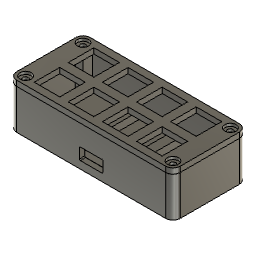
macropad v4 (Autodesk Fusion 360 design; units mm, degrees)
Autodesk Fusion 360 part; units mm, degrees
sketch "Sketch1" plane through (0, 0, 0) normal (0, 0, 1) x (1, 0, 0)
  line L0 (0, 1.7577) -> (18, 1.7577)
  line L1 (18, 1.7577) -> (18, -32.1423)
  line L2 (18, -32.1423) -> (0, -32.1423)
  line L3 (0, -32.1423) -> (0, 1.7577)
  line L4 (4.4, 2.6577) -> (13.6, 2.6577)
  line L5 (13.6, 2.6577) -> (13.6, -4.8423)
  line L6 (13.6, -4.8423) -> (4.4, -4.8423)
  line L7 (4.4, -4.8423) -> (4.4, 2.6577)
  dimension "d1" = 18
  dimension "d2" = 33.9
  dimension "d3" = 9.2
  dimension "d4" = 7.5
  dimension "d5" = 0.9
  dimension "d6" = 4.4
  dimension "d7" = 4.4
  constraint horizontal L0
  constraint vertical L1
  constraint horizontal L2
  constraint vertical L3
  constraint horizontal L4
  constraint vertical L5
  constraint horizontal L6
  constraint vertical L7
  measures "d1" distance of L0.start L0.end
  measures "d2" distance of L0.start L2.end
  measures "d3" distance of L4.start L4.end
  measures "d4" distance of L4.start L6.end
  measures "d5" distance of L0 L4
  measures "d6" distance of L1 L5
  measures "d7" distance of L3 L7
extrude "Extrude1" add sketch "Sketch1" against normal blind 1.75 contours L0 L1 L2 L3 L5 L6 L7 | L0 L5 L6 L7 makes body 1
extrude "Extrude2" add sketch "Sketch1" along normal blind 3.2 contours L0 L4 L5 L7 | L0 L5 L6 L7 bodies 1
fillet "Fillet1" radius 1 2 edges at (13.6, -1.0923, 3.2) (4.4, -1.0923, 3.2) on bodies 1
fillet "Fillet2" radius 1 2 edges at (13.6, 2.2077, 0) (4.4, 2.2077, 0) on bodies 1
sketch "Sketch2" plane through (0, 0, 0) normal (0, 0, 1) x (1, 0, 0)
  line L0 (0, 0) -> (-15.86, 0)
  line L1 (-15.86, 0) -> (-15.86, 15.86)
  line L2 (-15.86, 15.86) -> (0, 15.86)
  line L3 (0, 15.86) -> (0, 0)
  line L4 (-0.88, 14.98) -> (-14.98, 14.98)
  line L5 (-14.98, 14.98) -> (-14.98, 0.88)
  line L6 (-14.98, 0.88) -> (-0.88, 0.88)
  line L7 (-0.88, 0.88) -> (-0.88, 14.98)
  line L8 (-0.88, 14.98) -> (-14.98, 0.88) construction
  line L9 (-14.98, 14.98) -> (-0.88, 0.88) construction
  point P0 (-7.93, 7.93)
  dimension "d16" = 15.86
  dimension "d17" = 15.86
  dimension "d18" = 14.1
  dimension "d19" = 14.1
  dimension "d26" = 0.88
  dimension "d27" = 0.88
  dimension "d28" = 0.88
  dimension "d29" = 0.88
  constraint horizontal L0
  constraint vertical L1
  constraint horizontal L2
  constraint vertical L3
  constraint coincident L0.start L3.end
  constraint horizontal L4
  constraint perpendicular L4 L5
  constraint parallel L4 L6
  constraint parallel L5 L7
  constraint coincident L8 P0
  constraint coincident L9 P0
  measures "d16" distance of L0.start L0.end
  measures "d17" distance of L0.start L2.end
  measures "d18" distance of L5.end L6.end
  measures "d19" distance of L4.end L5.end
  measures "d26" distance of L1 L5
  measures "d27" distance of L3 L7
  measures "d28" distance of L0 L6
  measures "d29" distance of L2 L4
extrude "Extrude3" add sketch "Sketch2" along normal blind 1 separate body contours L0 L1 L2 L3 | L4 L5 L6 L7 makes body 2
extrude "Extrude4" add sketch "Sketch2" against normal blind 6 contours L4 L5 L6 L7 bodies 2
extrude "Extrude5" add sketch "Sketch2" along normal blind 5.5 contours L4 L5 L6 L7 bodies 2
extrude "Extrude6" cut 1 faces at (-10.28, 10.28, -6) along direction (0, 0, 1) blind 1 on bodies 2 bodies 2
sketch "Sketch3" plane through (0, 0, -5) normal (0, 0, -1) x (1, 0, 0)
  line L0 (-0.88, -14.98) -> (-0.88, -0.88)
  line L1 (-0.88, -0.88) -> (-14.98, -0.88)
  line L2 (-14.98, -0.88) -> (-14.98, -14.98)
  line L3 (-14.98, -14.98) -> (-0.88, -14.98)
  line L4 (-15.2053, -1.65) -> (-0.7947, -1.65)
  line L5 (-0.7947, -1.65) -> (-0.7947, -14.35)
  line L6 (-0.7947, -14.35) -> (-15.2053, -14.35)
  line L7 (-15.2053, -14.35) -> (-15.2053, -1.65)
  line L8 (-15.2053, -1.65) -> (-0.7947, -14.35) construction
  line L9 (-0.7947, -1.65) -> (-15.2053, -14.35) construction
  point P0 (-8, -8)
  dimension "d32" = 12.7
  constraint horizontal L4
  constraint perpendicular L4 L5
  constraint parallel L4 L6
  constraint parallel L5 L7
  constraint coincident L8 P0
  constraint coincident L9 P0
  measures "d32" distance of L4.end L5.end
sketch "Sketch5" plane through (-0.88, 0, 0) normal (1, 0, 0) x (0, 1, 0)
  line L0 (0.88, -5) -> (14.98, -5)
  line L1 (14.98, -5) -> (14.98, 0)
  line L2 (14.98, 0) -> (0.88, 0)
  line L3 (0.88, 0) -> (0.88, -5)
  line L4 (1.6501, -5) -> (0.88, 0)
  line L5 (14.3504, -5) -> (14.98, 0)
  constraint coincident L0 L4.start
  constraint coincident L2.end L3.start
  constraint coincident L0 L5.start
  constraint coincident L1.end L2.start
extrude "Extrude7" cut sketch "Sketch5" against normal blind 16 contours L0 L3 L4 | L0 L1 L5 bodies 2
sketch "Sketch7" plane through (0, 0, 5.5) normal (0, 0, 1) x (-1, 0, 0)
  line L0 (0.88, -0.88) -> (0.88, -14.98)
  line L1 (0.88, -14.98) -> (14.98, -14.98)
  line L2 (14.98, -14.98) -> (14.98, -0.88)
  line L3 (14.98, -0.88) -> (0.88, -0.88)
  line L4 (0.88, -12.98) -> (10.98, -12.98)
  line L5 (10.98, -12.98) -> (10.98, -2.88)
  line L6 (10.98, -2.88) -> (0.88, -2.88)
  line L7 (0.88, -2.88) -> (0.88, -12.98)
  line L8 (10.98, -2.88) -> (0.88, -2.88)
  line L9 (0.88, -2.88) -> (0.88, -0.88)
  line L10 (0.88, -0.88) -> (10.98, -0.88)
  line L11 (10.98, -0.88) -> (10.98, -2.88)
  dimension "d37" = 10.1
  dimension "d38" = 10.1
  dimension "d39" = 2
  dimension "d40" = 2
  constraint horizontal L4
  constraint vertical L5
  constraint horizontal L6
  constraint vertical L7
  constraint coincident L0 L4.start
  constraint horizontal L8
  constraint vertical L9
  constraint horizontal L10
  constraint vertical L11
  constraint coincident L0.start L3.end
  measures "d37" distance of L4.start L4.end
  measures "d38" distance of L4.start L6.end
  measures "d39" distance of L3 L6
  measures "d40" distance of L1 L4
sketch "Sketch8" plane through (-0.88, 0, 0) normal (1, 0, 0) x (0, 1, 0)
  line L0 (0.88, 1) -> (14.98, 1)
  line L1 (14.98, 1) -> (14.98, 5.5)
  line L2 (14.98, 5.5) -> (0.88, 5.5)
  line L3 (0.88, 5.5) -> (0.88, 1)
  line L4 (0.88, 1) -> (2.8805, 5.5)
  line L5 (14.98, 1) -> (13, 5.5)
  constraint coincident L0.start L3.end
  constraint coincident L2 L4.end
  constraint coincident L0.end L1.start
  constraint coincident L2 L5.end
extrude "Extrude8" cut sketch "Sketch8" against normal blind 17 contours L2 L3 L4 | L1 L2 L5 bodies 2
sketch "Sketch9" plane through (0, 12.9189, 5.6843) normal (0, 0.915315, 0.402739) x (-1, 0, 0)
  line L0 (14.98, -5.1177) -> (14.98, -0.2014)
  line L1 (14.98, -0.2014) -> (0.88, -0.2014)
  line L2 (0.88, -0.2014) -> (0.88, -5.1177)
  line L3 (0.88, -5.1177) -> (14.98, -5.1177)
  line L4 (10.98, -0.2014) -> (14.98, -5.1177)
  constraint coincident L1 L4.start
  constraint coincident L0.start L3.end
sketch "Sketch10" plane through (0, 0.3636, -0.1616) normal (0, -0.913774, 0.406224) x (1, 0, 0)
  line L0 (-14.98, 6.1959) -> (-14.98, 1.2713)
  line L1 (-14.98, 1.2713) -> (-0.88, 1.2713)
  line L2 (-0.88, 1.2713) -> (-0.88, 6.1959)
  line L3 (-0.88, 6.1959) -> (-14.98, 6.1959)
  line L4 (-10.9797, 6.1959) -> (-14.98, 1.2713)
  constraint coincident L3 L4.start
  constraint coincident L0.end L1.start
sketch "Sketch11" plane through (-14.98, 0, 0) normal (-1, 0, 0) x (0, -1, 0)
  line L0 (-0.88, 1) -> (-2.8805, 5.5)
  line L1 (-2.8805, 5.5) -> (-13, 5.5)
  line L2 (-13, 5.5) -> (-14.98, 1)
  line L3 (-14.98, 1) -> (-0.88, 1)
  line L4 (-0.88, 1) -> (-14.98, 1)
  constraint coincident L0.start L3.end
  constraint coincident L2.end L3.start
sketch "Sketch12" plane through (0, 0, 0) normal (0, 1, 0) x (1, 0, 0)
  line L0 (-15, -1) -> (-0.88, -1)
  line L1 (-0.88, -1) -> (-0.88, -5.5)
  line L2 (-0.88, -5.5) -> (-15, -5.5)
  line L3 (-15, -5.5) -> (-15, -1)
  constraint horizontal L0
  constraint vertical L1
  constraint horizontal L2
  constraint vertical L3
extrude "Extrude9" add sketch "Sketch12" along normal blind 3.3 bodies 2
sketch "Sketch13" plane through (0, 0, 5.5) normal (0, 0, 1) x (-1, 0, 0)
  line L0 (0.88, 0) -> (0.88, -13)
  line L1 (0.88, -13) -> (14.98, -13)
  line L2 (14.98, -13) -> (14.98, -3.3)
  line L3 (14.98, -3.3) -> (15, -3.3)
  line L4 (15, -3.3) -> (15, 0)
  line L5 (15, 0) -> (0.88, 0)
  line L6 (11, -0.9) -> (0.88, -0.9)
  line L7 (0.88, -0.9) -> (0.88, 0)
  line L8 (0.88, 0) -> (11, 0)
  line L9 (11, 0) -> (11, -0.9)
  constraint horizontal L6
  constraint vertical L7
  constraint horizontal L8
  constraint vertical L9
  constraint coincident L0.start L5.end
sketch "Sketch14" plane through (0, 0, 0) normal (0, -1, 0) x (1, 0, 0)
  line L0 (-15.86, 0) -> (0, 0)
  line L1 (0, 0) -> (0, 1)
  line L2 (0, 1) -> (-0.88, 1)
  line L3 (-0.88, 1) -> (-0.88, 5.5)
  line L4 (-0.88, 5.5) -> (-15, 5.5)
  line L5 (-15, 5.5) -> (-15, 1)
  line L6 (-15, 1) -> (-15.86, 1)
  line L7 (-15.86, 1) -> (-15.86, 0)
  line L8 (-15, 1) -> (-10.9774, 5.5)
  constraint coincident L5.end L6.start
  constraint coincident L4 L8.end
extrude "Extrude10" cut sketch "Sketch14" against normal blind 16 contours L4 L5 L8 bodies 2
sketch "Sketch15" plane through (-0.88, 7.93, 3.25) normal (1, 0, 0) x (0, 1, 0)
sketch "Sketch16" plane through (-0.88, 0, 0) normal (1, 0, 0) x (0, 1, 0)
  line L0 (0, 1) -> (14.98, 1)
  line L1 (14.98, 1) -> (13, 5.5)
  line L2 (13, 5.5) -> (0, 5.5)
  line L3 (0, 5.5) -> (0, 1)
  line L4 (0.8999, 5.5) -> (-1, 5.5)
  line L5 (-1, 5.5) -> (-1, 1)
  line L6 (-1, 1) -> (0.8999, 1)
  line L7 (0.8999, 1) -> (0.8999, 5.5)
  constraint horizontal L4
  constraint vertical L5
  constraint horizontal L6
  constraint vertical L7
  constraint coincident L2 L4.start
extrude "Extrude11" cut sketch "Sketch16" against normal blind 15 contours L0 L2 L3 L4 L6 L7 bodies 2
extrude "Extrude12" cut sketch "Sketch8" against normal blind 16.5 contours L2 L3 L4 bodies 2
fillet "Fillet3" radius 1.5 1 edges at (-0.88, 7.9403, 5.5) on bodies 2
sketch "Sketch17" plane through (0, 0, 0) normal (0, 0, 1) x (1, 0, 0)
  line L0 (45.22, -20.36) -> (-45.22, -20.36)
  line L1 (-45.22, -20.36) -> (-45.22, 20.36)
  line L2 (-45.22, 20.36) -> (45.22, 20.36)
  line L3 (45.22, 20.36) -> (45.22, -20.36)
  line L4 (45.22, -20.36) -> (-45.22, 20.36) construction
  line L5 (-45.22, -20.36) -> (45.22, 20.36) construction
  line L6 (-36.22, 17.36) -> (-20.36, 17.36)
  line L7 (-20.36, 17.36) -> (-20.36, 1.5)
  line L8 (-20.36, 1.5) -> (-36.22, 1.5)
  line L9 (-36.22, 1.5) -> (-36.22, 17.36)
  line L10 (-35.34, 16.48) -> (-21.24, 16.48)
  line L11 (-21.24, 16.48) -> (-21.24, 2.38)
  line L12 (-21.24, 2.38) -> (-35.34, 2.38)
  line L13 (-35.34, 2.38) -> (-35.34, 16.48)
  line L14 (-1.5, 17.36) -> (-1.5, 1.5)
  line L15 (-2.38, 16.48) -> (-2.38, 2.38)
  line L16 (-2.38, 2.38) -> (-16.48, 2.38)
  line L17 (-1.5, 1.5) -> (-17.36, 1.5)
  line L18 (-17.36, 1.5) -> (-17.36, 17.36)
  line L19 (-16.48, 2.38) -> (-16.48, 16.48)
  line L20 (-17.36, 17.36) -> (-1.5, 17.36)
  line L21 (-16.48, 16.48) -> (-2.38, 16.48)
  line L22 (17.36, 17.36) -> (17.36, 1.5)
  line L23 (16.48, 16.48) -> (16.48, 2.38)
  line L24 (16.48, 2.38) -> (2.38, 2.38)
  line L25 (17.36, 1.5) -> (1.5, 1.5)
  line L26 (1.5, 1.5) -> (1.5, 17.36)
  line L27 (2.38, 2.38) -> (2.38, 16.48)
  line L28 (1.5, 17.36) -> (17.36, 17.36)
  line L29 (2.38, 16.48) -> (16.48, 16.48)
  line L30 (36.22, 17.36) -> (36.22, 1.5)
  line L31 (35.34, 16.48) -> (35.34, 2.38)
  line L32 (35.34, 2.38) -> (21.24, 2.38)
  line L33 (36.22, 1.5) -> (20.36, 1.5)
  line L34 (20.36, 1.5) -> (20.36, 17.36)
  line L35 (21.24, 2.38) -> (21.24, 16.48)
  line L36 (20.36, 17.36) -> (36.22, 17.36)
  line L37 (21.24, 16.48) -> (35.34, 16.48)
  line L38 (-36.22, -17.36) -> (-36.22, -1.5)
  line L39 (-35.34, -16.48) -> (-35.34, -2.38)
  line L40 (-36.22, -1.5) -> (-20.36, -1.5)
  line L41 (-35.34, -2.38) -> (-21.24, -2.38)
  line L42 (-20.36, -1.5) -> (-20.36, -17.36)
  line L43 (-21.24, -2.38) -> (-21.24, -16.48)
  line L44 (-21.24, -16.48) -> (-35.34, -16.48)
  line L45 (-20.36, -17.36) -> (-36.22, -17.36)
  line L46 (-1.5, -17.36) -> (-17.36, -17.36)
  line L47 (-2.38, -16.48) -> (-16.48, -16.48)
  line L48 (-16.48, -16.48) -> (-16.48, -2.38)
  line L49 (-17.36, -17.36) -> (-17.36, -1.5)
  line L50 (-17.36, -1.5) -> (-1.5, -1.5)
  line L51 (-16.48, -2.38) -> (-2.38, -2.38)
  line L52 (-1.5, -1.5) -> (-1.5, -17.36)
  line L53 (-2.38, -2.38) -> (-2.38, -16.48)
  line L54 (1.5, -17.36) -> (1.5, -1.5)
  line L55 (2.38, -16.48) -> (2.38, -2.38)
  line L56 (2.38, -2.38) -> (16.48, -2.38)
  line L57 (1.5, -1.5) -> (17.36, -1.5)
  line L58 (16.48, -2.38) -> (16.48, -16.48)
  line L59 (17.36, -1.5) -> (17.36, -17.36)
  line L60 (16.48, -16.48) -> (2.38, -16.48)
  line L61 (17.36, -17.36) -> (1.5, -17.36)
  line L62 (36.22, -17.36) -> (20.36, -17.36)
  line L63 (35.34, -16.48) -> (21.24, -16.48)
  line L64 (20.36, -17.36) -> (20.36, -1.5)
  line L65 (21.24, -16.48) -> (21.24, -2.38)
  line L66 (21.24, -2.38) -> (35.34, -2.38)
  line L67 (20.36, -1.5) -> (36.22, -1.5)
  line L68 (35.34, -2.38) -> (35.34, -16.48)
  line L69 (36.22, -1.5) -> (36.22, -17.36)
  circle A0 centre (-40.72, 15.86) radius 3.125
  circle A1 centre (-40.72, -15.86) radius 3.125
  circle A2 centre (40.72, -15.86) radius 3.125
  circle A3 centre (40.72, 15.86) radius 3.125
  circle A4 centre (40.72, -15.86) radius 1.525
  circle A5 centre (40.72, 15.86) radius 1.525
  circle A6 centre (-40.72, 15.86) radius 1.525
  circle A7 centre (-40.72, -15.86) radius 1.525
  dimension "d53" = 90.44
  dimension "d54" = 40.72
  dimension "d55" = 15.86
  dimension "d56" = 15.86
  dimension "d57" = 14.1
  dimension "d58" = 14.1
  dimension "d59" = 0.88
  dimension "d60" = 0.88
  dimension "d61" = 0.88
  dimension "d62" = 0.88
  dimension "d63" = 9
  dimension "d64" = 3
  dimension "d65" = 15.86
  dimension "d66" = 15.86
  dimension "d67" = 14.1
  dimension "d68" = 14.1
  dimension "d69" = 0.88
  dimension "d70" = 0.88
  dimension "d71" = 0.88
  dimension "d72" = 0.88
  dimension "d73" = 15.86
  dimension "d74" = 15.86
  dimension "d75" = 14.1
  dimension "d76" = 14.1
  dimension "d77" = 0.88
  dimension "d78" = 0.88
  dimension "d79" = 0.88
  dimension "d80" = 0.88
  dimension "d81" = 15.86
  dimension "d82" = 15.86
  dimension "d83" = 14.1
  dimension "d84" = 14.1
  dimension "d85" = 0.88
  dimension "d86" = 0.88
  dimension "d87" = 0.88
  dimension "d88" = 0.88
  dimension "d89" = 3
  dimension "d90" = 3
  dimension "d91" = 3
  dimension "d92" = 9
  dimension "d93" = 3
  dimension "d94" = 3
  dimension "d95" = 3
  dimension "d96" = 15.86
  dimension "d97" = 15.86
  dimension "d98" = 14.1
  dimension "d99" = 14.1
  dimension "d100" = 0.88
  dimension "d101" = 0.88
  dimension "d102" = 0.88
  dimension "d103" = 0.88
  dimension "d104" = 15.86
  dimension "d105" = 15.86
  dimension "d106" = 14.1
  dimension "d107" = 14.1
  dimension "d108" = 0.88
  dimension "d109" = 0.88
  dimension "d110" = 0.88
  dimension "d111" = 0.88
  dimension "d112" = 15.86
  dimension "d113" = 15.86
  dimension "d114" = 14.1
  dimension "d115" = 14.1
  dimension "d116" = 0.88
  dimension "d117" = 0.88
  dimension "d118" = 0.88
  dimension "d119" = 0.88
  dimension "d120" = 15.86
  dimension "d121" = 15.86
  dimension "d122" = 14.1
  dimension "d123" = 14.1
  dimension "d124" = 0.88
  dimension "d125" = 0.88
  dimension "d126" = 0.88
  dimension "d127" = 0.88
  dimension "d128" = 3
  dimension "d129" = 3
  dimension "d130" = 3
  dimension "d131" = 3
  dimension "d132" = 3
  dimension "d133" = 3
  dimension "d134" = 3
  dimension "d135" = 6.25
  dimension "d136" = 4.5
  dimension "d137" = 4.5
  dimension "d138" = 6.25
  dimension "d139" = 6.25
  dimension "d140" = 6.25
  dimension "d141" = 4.5
  dimension "d142" = 4.5
  dimension "d143" = 4.5
  dimension "d144" = 4.5
  dimension "d145" = 4.5
  dimension "d146" = 4.5
  dimension "d147" = 3.05
  dimension "d148" = 3.05
  dimension "d149" = 3.05
  dimension "d150" = 3.05
  constraint horizontal L0
  constraint perpendicular L0 L1
  constraint parallel L0 L2
  constraint parallel L1 L3
  constraint coincident L4 origin
  constraint coincident L5 origin
  constraint horizontal L6
  constraint vertical L7
  constraint horizontal L8
  constraint vertical L9
  constraint horizontal L10
  constraint vertical L11
  constraint horizontal L12
  constraint vertical L13
  constraint horizontal L20
  constraint vertical L14
  constraint horizontal L17
  constraint vertical L18
  constraint horizontal L21
  constraint vertical L15
  constraint horizontal L16
  constraint vertical L19
  constraint horizontal L28
  constraint vertical L22
  constraint horizontal L25
  constraint vertical L26
  constraint horizontal L29
  constraint vertical L23
  constraint horizontal L24
  constraint vertical L27
  constraint horizontal L36
  constraint vertical L30
  constraint horizontal L33
  constraint vertical L34
  constraint horizontal L37
  constraint vertical L31
  constraint horizontal L32
  constraint vertical L35
  constraint horizontal L40
  constraint vertical L42
  constraint horizontal L45
  constraint vertical L38
  constraint horizontal L41
  constraint vertical L43
  constraint horizontal L44
  constraint vertical L39
  constraint horizontal L50
  constraint vertical L52
  constraint horizontal L46
  constraint vertical L49
  constraint horizontal L51
  constraint vertical L53
  constraint horizontal L47
  constraint vertical L48
  constraint horizontal L57
  constraint vertical L59
  constraint horizontal L61
  constraint vertical L54
  constraint horizontal L56
  constraint vertical L58
  constraint horizontal L60
  constraint vertical L55
  constraint horizontal L67
  constraint vertical L69
  constraint horizontal L62
  constraint vertical L64
  constraint horizontal L66
  constraint vertical L68
  constraint horizontal L63
  constraint vertical L65
  constraint concentric A2 A4
  constraint concentric A3 A5
  constraint concentric A0 A6
  constraint concentric A1 A7
  measures "d53" distance of L1.end L2.end
  measures "d54" distance of L0.end L1.end
  measures "d55" distance of L6.start L6.end
  measures "d56" distance of L6.start L8.end
  measures "d57" distance of L10.start L10.end
  measures "d58" distance of L10.start L12.end
  measures "d59" distance of L7 L11
  measures "d60" distance of L9 L13
  measures "d61" distance of L6 L10
  measures "d62" distance of L8 L12
  measures "d63" distance of L1 L9
  measures "d64" distance of L2 L6
  measures "d65" distance of L18.end L14.start
  measures "d66" distance of L18.end L17.end
  measures "d67" distance of L19.end L15.start
  measures "d68" distance of L16.end L19.end
  measures "d69" distance of L14 L15
  measures "d70" distance of L18 L19
  measures "d71" distance of L20 L21
  measures "d72" distance of L16 L17
  measures "d73" distance of L26.end L22.start
  measures "d74" distance of L26.end L25.end
  measures "d75" distance of L27.end L23.start
  measures "d76" distance of L24.end L27.end
  measures "d77" distance of L22 L23
  measures "d78" distance of L26 L27
  measures "d79" distance of L28 L29
  measures "d80" distance of L24 L25
  measures "d81" distance of L34.end L30.start
  measures "d82" distance of L34.end L33.end
  measures "d83" distance of L35.end L31.start
  measures "d84" distance of L32.end L35.end
  measures "d85" distance of L30 L31
  measures "d86" distance of L34 L35
  measures "d87" distance of L36 L37
  measures "d88" distance of L32 L33
  measures "d89" distance of L7 L18
  measures "d90" distance of L14 L26
  measures "d91" distance of L22 L34
  measures "d92" distance of L3 L30
  measures "d93" distance of L2 L20
  measures "d94" distance of L2 L28
  measures "d95" distance of L2 L36
  measures "d96" distance of L38.end L40.end
  measures "d97" distance of L38.end L38.start
  measures "d98" distance of L39.end L41.end
  measures "d99" distance of L39.start L39.end
  measures "d100" distance of L42 L43
  measures "d101" distance of L38 L39
  measures "d102" distance of L40 L41
  measures "d103" distance of L44 L45
  measures "d104" distance of L50.end L49.end
  measures "d105" distance of L46.end L49.end
  measures "d106" distance of L51.end L48.end
  measures "d107" distance of L47.end L48.end
  measures "d108" distance of L52 L53
  measures "d109" distance of L48 L49
  measures "d110" distance of L50 L51
  measures "d111" distance of L46 L47
  measures "d112" distance of L54.end L57.end
  measures "d113" distance of L54.end L54.start
  measures "d114" distance of L55.end L56.end
  measures "d115" distance of L55.start L55.end
  measures "d116" distance of L58 L59
  measures "d117" distance of L54 L55
  measures "d118" distance of L56 L57
  measures "d119" distance of L60 L61
  measures "d120" distance of L64.end L67.end
  measures "d121" distance of L64.end L62.end
  measures "d122" distance of L65.end L66.end
  measures "d123" distance of L65.end L63.end
  measures "d124" distance of L68 L69
  measures "d125" distance of L64 L65
  measures "d126" distance of L66 L67
  measures "d127" distance of L62 L63
  measures "d128" distance of L42 L49
  measures "d129" distance of L52 L54
  measures "d130" distance of L59 L64
  measures "d131" distance of L0 L45
  measures "d132" distance of L0 L46
  measures "d133" distance of L0 L61
  measures "d134" distance of L0 L62
  measures "d135" diameter of A0
  measures "d136" distance of L1 A0.centre
  measures "d137" distance of L2 A0.centre
  measures "d138" diameter of A1
  measures "d139" diameter of A2
  measures "d140" diameter of A3
  measures "d141" distance of L0 A1.centre
  measures "d142" distance of L1 A1.centre
  measures "d143" distance of L0 A2.centre
  measures "d144" distance of L3 A2.centre
  measures "d145" distance of L3 A3.centre
  measures "d146" distance of L2 A3.centre
  measures "d147" diameter of A4
  measures "d148" diameter of A5
  measures "d149" diameter of A6
  measures "d150" diameter of A7
sketch "Sketch18" plane through (0, 0, 0) normal (0, 0, 1) x (1, 0, 0)
  line L0 (-45.22, 20.36) -> (45.22, 20.36)
  line L1 (45.22, 20.36) -> (45.22, -20.36)
  line L2 (45.22, -20.36) -> (-45.22, -20.36)
  line L3 (-45.22, -20.36) -> (-45.22, 20.36)
  line L4 (-41.22, 17.36) -> (41.22, 17.36)
  line L5 (41.22, 17.36) -> (41.22, -17.36)
  line L6 (41.22, -17.36) -> (-41.22, -17.36)
  line L7 (-41.22, -17.36) -> (-41.22, 17.36)
  line L8 (-45.22, 20.36) -> (-36.97, 20.36)
  line L9 (-36.97, 20.36) -> (-36.97, 12.11)
  line L10 (-36.97, 12.11) -> (-45.22, 12.11)
  line L11 (-45.22, 12.11) -> (-45.22, 20.36)
  line L12 (-45.22, -20.36) -> (-36.97, -20.36)
  line L13 (-36.97, -20.36) -> (-36.97, -12.11)
  line L14 (-36.97, -12.11) -> (-45.22, -12.11)
  line L15 (-45.22, -12.11) -> (-45.22, -20.36)
  line L16 (45.22, -20.36) -> (36.97, -20.36)
  line L17 (36.97, -20.36) -> (36.97, -12.11)
  line L18 (36.97, -12.11) -> (45.22, -12.11)
  line L19 (45.22, -12.11) -> (45.22, -20.36)
  line L20 (45.22, 20.36) -> (36.97, 20.36)
  line L21 (36.97, 20.36) -> (36.97, 12.11)
  line L22 (36.97, 12.11) -> (45.22, 12.11)
  line L23 (45.22, 12.11) -> (45.22, 20.36)
  line L24 (-9, 16.95) -> (9, 16.95)
  line L25 (9, 16.95) -> (9, -16.95)
  line L26 (9, -16.95) -> (-9, -16.95)
  line L27 (-9, -16.95) -> (-9, 16.95)
  line L28 (-9, 16.95) -> (9, -16.95) construction
  line L29 (9, 16.95) -> (-9, -16.95) construction
  line L30 (4.6, -17.85) -> (-4.6, -17.85)
  line L31 (-4.6, -17.85) -> (-4.6, -7.85)
  line L32 (-4.6, -7.85) -> (4.6, -7.85)
  line L33 (4.6, -7.85) -> (4.6, -17.85)
  line L34 (4.6, -17.85) -> (-4.6, -7.85) construction
  line L35 (-4.6, -17.85) -> (4.6, -7.85) construction
  line L36 (8.4777, -14.36) -> (-8.4777, -14.36)
  line L37 (-8.4777, -14.36) -> (-8.4777, -26.36)
  line L38 (-8.4777, -26.36) -> (8.4777, -26.36)
  line L39 (8.4777, -26.36) -> (8.4777, -14.36)
  line L40 (8.4777, -14.36) -> (-8.4777, -26.36) construction
  line L41 (-8.4777, -14.36) -> (8.4777, -26.36) construction
  line L42 (9.5, 17.36) -> (14.5, 17.36)
  line L43 (14.5, 17.36) -> (14.5, -17.36)
  line L44 (14.5, -17.36) -> (9.5, -17.36)
  line L45 (9.5, -17.36) -> (9.5, 17.36)
  line L46 (-9.5, -17.36) -> (-14.5, -17.36)
  line L47 (-14.5, -17.36) -> (-14.5, 17.36)
  line L48 (-14.5, 17.36) -> (-9.5, 17.36)
  line L49 (-9.5, 17.36) -> (-9.5, -17.36)
  point P0 (0, -12.85)
  point P1 (0, -20.36)
  dimension "d151" = 4
  dimension "d152" = 3
  dimension "d153" = 4
  dimension "d154" = 3
  dimension "d155" = 8.25
  dimension "d156" = 8.25
  dimension "d157" = 8.25
  dimension "d158" = 8.25
  dimension "d159" = 8.25
  dimension "d160" = 8.25
  dimension "d161" = 8.25
  dimension "d162" = 8.25
  dimension "d163" = 18
  dimension "d164" = 33.9
  dimension "d165" = 9.2
  dimension "d166" = 10
  dimension "d167" = 0.9
  dimension "d168" = 12
  dimension "d169" = 5
  dimension "d170" = 5
  dimension "d171" = 0.5
  dimension "d172" = 0.5
  constraint horizontal L0
  constraint vertical L1
  constraint horizontal L2
  constraint vertical L3
  constraint horizontal L4
  constraint vertical L5
  constraint horizontal L6
  constraint vertical L7
  constraint horizontal L8
  constraint vertical L9
  constraint horizontal L10
  constraint vertical L11
  constraint horizontal L12
  constraint vertical L13
  constraint horizontal L14
  constraint vertical L15
  constraint horizontal L16
  constraint vertical L17
  constraint horizontal L18
  constraint vertical L19
  constraint horizontal L20
  constraint vertical L21
  constraint horizontal L22
  constraint vertical L23
  constraint horizontal L24
  constraint perpendicular L24 L25
  constraint parallel L24 L26
  constraint parallel L25 L27
  constraint coincident L28 origin
  constraint coincident L29 origin
  constraint horizontal L30
  constraint perpendicular L30 L31
  constraint parallel L30 L32
  constraint parallel L31 L33
  constraint coincident L34 P0
  constraint coincident L35 P0
  constraint horizontal L36
  constraint perpendicular L36 L37
  constraint parallel L36 L38
  constraint parallel L37 L39
  constraint coincident L40 P1
  constraint coincident L41 P1
  constraint midpoint L2 P1
  constraint horizontal L42
  constraint vertical L43
  constraint horizontal L44
  constraint vertical L45
  constraint coincident L6 L43.end
  constraint coincident L4 L42.start
  constraint horizontal L46
  constraint vertical L47
  constraint horizontal L48
  constraint vertical L49
  constraint coincident L6 L46.start
  measures "d151" distance of L3 L7
  measures "d152" distance of L0 L4
  measures "d153" distance of L1 L5
  measures "d154" distance of L2 L6
  measures "d155" distance of L0.start L8.end
  measures "d156" distance of L0.start L10.end
  measures "d157" distance of L2.end L12.end
  measures "d158" distance of L2.end L14.end
  measures "d159" distance of L1.end L16.end
  measures "d160" distance of L1.end L18.end
  measures "d161" distance of L0.end L20.end
  measures "d162" distance of L0.end L22.end
  measures "d163" distance of L25.end L26.end
  measures "d164" distance of L24.end L25.end
  measures "d165" distance of L31.end L32.end
  measures "d166" distance of L30.end L31.end
  measures "d167" distance of L26 L30
  measures "d168" distance of L36.end L37.end
  measures "d169" distance of L43 L45
  measures "d170" distance of L47 L49
  measures "d171" distance of L27 L49
  measures "d172" distance of L25 L45
extrude "Extrude13" add sketch "Sketch18" against normal blind 4 separate body contours L0 L3 L4 L7 L8 L9 L10 L11 | L0 L4 L9 L21 L42 L48 | L3 L7 L10 L14 | L0 L1 L4 L5 L20 L21 L22 L23 | L4 L7 L9 L10 | L4 L6 L7 L9 L10 L13 L14 L47 | L2 L3 L6 L7 L12 L13 L14 L15 | L4 L5 L6 L17 L18 L21 L22 L43 | L4 L5 L21 L22 | L4 L6 L46 L47 L48 L49 | L6 L7 L13 L14 | L1 L5 L18 L22 | L4 L6 L42 L43 L44 L45 | L4 L6 L24 L25 L26 L27 L37 L39 L45 L49 | L2 L6 L13 L37 L46 | L1 L2 L5 L6 L16 L17 L18 L19 | L2 L6 L17 L39 L44 | L2 L6 L30 L31 L33 L37 L39 | L5 L6 L17 L18 | L6 L26 L31 L37 | L6 L26 L33 L39 | L6 L26 L31 L33 | L6 L30 L31 L33 | L26 L31 L36 L37 | L24 L25 L26 L27 L31 L32 L33 L36 L37 L39 | L26 L33 L36 L39 | L26 L31 L33 L36 | L31 L32 L33 L36 makes body 3
extrude "Extrude14" add sketch "Sketch18" along normal blind 18 contours L0 L3 L4 L7 L8 L9 L10 L11 | L0 L4 L9 L21 L42 L48 | L3 L7 L10 L14 | L0 L1 L4 L5 L20 L21 L22 L23 | L4 L7 L9 L10 | L2 L3 L6 L7 L12 L13 L14 L15 | L4 L5 L21 L22 | L6 L7 L13 L14 | L1 L5 L18 L22 | L2 L6 L13 L37 L46 | L1 L2 L5 L6 L16 L17 L18 L19 | L2 L6 L17 L39 L44 | L2 L6 L30 L31 L33 L37 L39 | L5 L6 L17 L18 | L6 L30 L31 L33 bodies 3
extrude "Extrude15" add sketch "Sketch18" along normal blind 1.75 separate body contours L24 L25 L26 L27 L31 L32 L33 L36 L37 L39 makes body 4
extrude "Extrude16" add sketch "Sketch18" along normal blind 1.75 contours L26 L31 L36 L37 | L26 L33 L36 L39 bodies 4
extrude "Extrude17" add sketch "Sketch18" along normal blind 4.95 contours L6 L26 L31 L33 | L6 L30 L31 L33 | L26 L31 L33 L36 | L31 L32 L33 L36 bodies 4
sketch "Sketch19" plane through (0, -17.85, 0) normal (0, -1, 0) x (1, 0, 0)
  line L0 (-4.6, 0) -> (4.6, 0)
  line L1 (4.6, 0) -> (4.6, 4.95)
  line L2 (4.6, 4.95) -> (-4.6, 4.95)
  line L3 (-4.6, 4.95) -> (-4.6, 0)
  line L4 (-4.6, 1.749) -> (4.6, 1.749)
  line L5 (4.6, 1.749) -> (4.6, 0)
  line L6 (4.6, 0) -> (-4.6, 0)
  line L7 (-4.6, 0) -> (-4.6, 1.749)
  constraint horizontal L4
  constraint vertical L5
  constraint horizontal L6
  constraint vertical L7
  constraint coincident L0.end L1.start
  constraint coincident L3 L4.start
extrude "Extrude18" cut sketch "Sketch19" against normal blind 0.9 contours L0 L1 L3 L4 L5 L6 L7 bodies 4
extrude "Extrude19" add sketch "Sketch18" along normal blind 4 contours L4 L6 L46 L47 L48 L49 | L4 L6 L42 L43 L44 L45 bodies 3
sketch "Sketch20" plane through (0, -20.36, 0) normal (0, -1, 0) x (1, 0, 0)
  line L0 (-45.22, 18) -> (-45.22, -4)
  line L1 (-45.22, -4) -> (45.22, -4)
  line L2 (45.22, -4) -> (45.22, 18)
  line L3 (45.22, 18) -> (-45.22, 18)
  line L4 (-6.5, 6.6) -> (6.5, 6.6)
  line L5 (6.5, 6.6) -> (6.5, 0.1)
  line L6 (6.5, 0.1) -> (-6.5, 0.1)
  line L7 (-6.5, 0.1) -> (-6.5, 6.6)
  line L8 (-6.5, 6.6) -> (6.5, 0.1) construction
  line L9 (6.5, 6.6) -> (-6.5, 0.1) construction
  point P0 (0, 3.35)
  dimension "d187" = 13
  dimension "d188" = 6.5
  constraint horizontal L4
  constraint perpendicular L4 L5
  constraint parallel L4 L6
  constraint parallel L5 L7
  constraint coincident L8 P0
  constraint coincident L9 P0
  measures "d187" distance of L5.end L6.end
  measures "d188" distance of L4.end L5.end
extrude "Extrude20" cut sketch "Sketch20" against normal blind 4 contours L4 L5 L6 L7 bodies 3
fillet "Fillet4" radius 0.5 4 edges at (-6.5, -18.86, 0.1) (-6.5, -18.86, 6.6) (6.5, -18.86, 6.6) (6.5, -18.86, 0.1) on bodies 3
move_body "Move1" bodies 3 to x (1, 0, 0) y (0, 1, 0) z (0, 0, 1) at (0, 0, -30)
move_body "Move2" bodies 3 to x (1, 0, 0) y (0, 1, 0) z (0, 0, 1) at (0, 0, -2)
extrude "Extrude21" add sketch "Sketch17" against normal blind 3 separate body contours L0 L1 L2 L3 | L6 L7 L8 L9 | L14 L17 L18 L20 | L22 L25 L26 L28 | L30 L33 L34 L36 | L38 L40 L42 L45 | L46 L49 L50 L52 | L54 L57 L59 L61 | L62 L64 L67 L69 | A0 | A1 | A2 | A3 makes body 5
move_body "Move3" bodies 4 to x (1, 0, 0) y (0, 1, 0) z (0, 0, 1) at (0, 0, -32)
move_body "Move4" bodies 5 to x (1, 0, 0) y (0, 1, 0) z (0, 0, 1) at (0, 0, -11)
fillet "Fillet5" radius 4 4 edges at (45.22, -20.36, -12.5) (45.22, 20.36, -12.5) (-45.22, 20.36, -12.5) (-45.22, -20.36, -12.5) on bodies 5
fillet "Fillet6" radius 4 1 edges at (-45.22, -20.36, -25) on bodies 3
fillet "Fillet7" radius 4 3 edges at (-45.22, 20.36, -25) (45.22, 20.36, -25) (45.22, -20.36, -25) on bodies 3
move_body "Move5" bodies 5 to x (1, 0, 0) y (0, 1, 0) z (0, 0, 1) at (0, 0, 11)
extrude "Extrude22" cut sketch "Sketch17" against normal blind 1.5 contours A0 | A1 | A2 | A3 bodies 5
move_body "Move6" bodies 3 to x (1, 0, 0) y (0, 1, 0) z (0, 0, 1) at (0, 0, 14)
sketch "Sketch21" plane through (0, 0, 0) normal (0, 0, 1) x (-1, 0, 0)
  line L0 (36.97, -12.11) -> (36.97, -17.36)
  line L1 (36.97, -17.36) -> (-36.97, -17.36)
  line L2 (-36.97, -17.36) -> (-36.97, -12.11)
  line L3 (-36.97, -12.11) -> (-41.22, -12.11)
  line L4 (-41.22, -12.11) -> (-41.22, 12.11)
  line L5 (-41.22, 12.11) -> (-36.97, 12.11)
  line L6 (-36.97, 12.11) -> (-36.97, 17.36)
  line L7 (-36.97, 17.36) -> (36.97, 17.36)
  line L8 (36.97, 17.36) -> (36.97, 12.11)
  line L9 (36.97, 12.11) -> (41.22, 12.11)
  line L10 (41.22, 12.11) -> (41.22, -12.11)
  line L11 (41.22, -12.11) -> (36.97, -12.11)
  arc A0 (-41.22, 20.36) -> (-45.22, 16.36) centre (-41.22, 16.36) ccw
  line L12 (-45.22, 16.36) -> (-45.22, -16.36)
  arc A1 (-45.22, -16.36) -> (-41.22, -20.36) centre (-41.22, -16.36) ccw
  line L13 (-41.22, -20.36) -> (41.22, -20.36)
  arc A2 (41.22, -20.36) -> (45.22, -16.36) centre (41.22, -16.36) ccw
  line L14 (45.22, -16.36) -> (45.22, 16.36)
  arc A3 (45.22, 16.36) -> (41.22, 20.36) centre (41.22, 16.36) ccw
  line L15 (41.22, 20.36) -> (-41.22, 20.36)
  line L16 (39.1009, -13.0615) -> (37.4868, -15.863)
  line L17 (37.4868, -15.863) -> (39.106, -18.6615)
  line L18 (39.106, -18.6615) -> (42.3391, -18.6585)
  line L19 (42.3391, -18.6585) -> (43.9532, -15.857)
  line L20 (43.9532, -15.857) -> (42.334, -13.0585)
  line L21 (42.334, -13.0585) -> (39.1009, -13.0615)
  line L22 (37.92, 14.2434) -> (40.72, 12.6268)
  line L23 (40.72, 12.6268) -> (43.52, 14.2434)
  line L24 (43.52, 14.2434) -> (43.52, 17.4766)
  line L25 (43.52, 17.4766) -> (40.72, 19.0932)
  line L26 (40.72, 19.0932) -> (37.92, 17.4766)
  line L27 (37.92, 17.4766) -> (37.92, 14.2434)
  line L28 (-37.92, 17.4766) -> (-40.72, 19.0932)
  line L29 (-40.72, 19.0932) -> (-43.52, 17.4766)
  line L30 (-43.52, 17.4766) -> (-43.52, 14.2434)
  line L31 (-43.52, 14.2434) -> (-40.72, 12.6268)
  line L32 (-40.72, 12.6268) -> (-37.92, 14.2434)
  line L33 (-37.92, 14.2434) -> (-37.92, 17.4766)
  line L34 (-37.92, -14.2434) -> (-40.72, -12.6268)
  line L35 (-40.72, -12.6268) -> (-43.52, -14.2434)
  line L36 (-43.52, -14.2434) -> (-43.52, -17.4766)
  line L37 (-43.52, -17.4766) -> (-40.72, -19.0932)
  line L38 (-40.72, -19.0932) -> (-37.92, -17.4766)
  line L39 (-37.92, -17.4766) -> (-37.92, -14.2434)
  point P0 (40.72, -15.86)
  point P1 (40.72, 15.86)
  point P2 (-40.72, 15.86)
  point P3 (-40.72, -15.86)
  dimension "d203" = 2.8
  dimension "d204" = 2.8
  dimension "d205" = 2.8
  dimension "d206" = 2.8
  measures "d203" distance of P0 L21
  measures "d204" distance of P1 L27
  measures "d205" distance of P2 L33
  measures "d206" distance of P3 L39
extrude "Extrude23" cut sketch "Sketch21" against normal blind 17 contours L16 L17 L18 L19 L20 L21 | L22 L23 L24 L25 L26 L27 | L28 L29 L30 L31 L32 L33 | L34 L35 L36 L37 L38 L39 bodies 3
extrude "Extrude24" add 4 faces at (-41.258, 14.9262, -17) (-41.6533, -16.3989, -17) (41.6533, -15.3211, -17) (41.6533, 16.3989, -17) along direction (0, 0, 1) blind 8 on bodies 3 bodies 3
extrude "Extrude25" add 4 faces at (-41.6533, -16.3989, -9) (41.6533, -15.3211, -9) (41.6533, 16.3989, -9) (-41.258, 14.9262, -9) along direction (0, 0, 1) blind 2.4 separate body on bodies 3 makes body 6 at (41.6533, 16.3989, -9) makes body 7 at (-41.6533, -16.3989, -9) makes body 8 at (41.6533, -15.3211, -9) makes body 9 at (-41.258, 14.9262, -9)
extrude "Extrude26" add 4 faces at (41.6533, 16.3989, -6.6) (41.6533, -15.3211, -6.6) (-41.6533, -16.3989, -6.6) (-41.258, 14.9262, -6.6) along direction (0, 0, 1) blind 6.6 separate body on bodies 6 7 8 9 makes body 10 at (-41.6533, -16.3989, -6.6) makes body 11 at (41.6533, 16.3989, -6.6) makes body 12 at (41.6533, -15.3211, -6.6) makes body 13 at (-41.258, 14.9262, -6.6)
combine "Combine1" operation add target body 3 tool bodies 10 11 12 13
extrude "Extrude27" cut sketch "Sketch17" against normal blind 15 contours A4 | A5 | A6 | A7 bodies 3
move_body "Move7" bodies 5 to x (1, 0, 0) y (0, 1, 0) z (0, 0, 1) at (0, 0, 3)
move_body "Move8" bodies 2 to x (1, 0, 0) y (0, 1, 0) z (0, 0, 1) at (-1, 0, 3)
hidden bodies 1 2 4 6 7 8 9
